remote_holder (Autodesk Fusion 360 design; units mm, degrees)
Autodesk Fusion 360 part; units mm, degrees
sketch "Sketch1" plane through (0, 0, 0) normal (0, 0, 1) x (1, 0, 0)
  line L0 (0, 0) -> (-42, 0)
  line L1 (-42, 0) -> (-42, 10)
  line L2 (-42, 10) -> (0, 10)
  line L3 (0, 10) -> (0, 0)
  line L4 (3.6, -3.6) -> (-45.6, -3.6)
  line L5 (-45.6, -3.6) -> (-45.6, 13.6)
  line L6 (-45.6, 13.6) -> (3.6, 13.6)
  line L7 (3.6, 13.6) -> (3.6, -3.6)
  dimension "d1" = 42
  dimension "d2" = 10
  dimension "d3" = -3.6
  constraint horizontal L0
  constraint vertical L1
  constraint horizontal L2
  constraint vertical L3
  constraint coincident L0.start L3.end
  measures "d1" distance of L0.start L0.end
  measures "d2" distance of L0.start L2.end
extrude "Extrude1" add sketch "Sketch1" along normal blind 65
extrude "Extrude2" add sketch "Sketch1" against normal blind 5 contours L0 L1 L2 L3 | L4 L5 L6 L7
sketch "Sketch2" plane through (0, -3.6, 0) normal (0, -1, 0) x (1, 0, 0)
  line L0 (3.6, -5) -> (3.6, 65)
  line L1 (3.6, 65) -> (-45.6, 65)
  line L2 (-45.6, 65) -> (-45.6, -5)
  line L3 (-45.6, -5) -> (3.6, -5)
  line L4 (0, 65, -3.6) -> (0, 65, 0)
  line L5 (-42, 65, -3.6) -> (-42, 65, 0)
  line L6 (-21, 65) -> (-21, -5)
  spline S0 degree 2 poles (-42, 65) (-21, 34) (0, 65) knots 0 0 0 5.982089 5.982089 5.982089 weights 1 2.19545 1
  point P0 (0, 65)
  point P1 (-42, 65)
  constraint coincident P0 S0.end
  constraint coincident L1 P0
  constraint coincident P1 S0.start
  constraint coincident L1 P1
  constraint midpoint L1 L6.start
  constraint midpoint L3 L6.end
extrude "Extrude3" cut sketch "Sketch2" against normal blind 13.6 contours L1 L6 S0 | L1 L6 S0
fillet "Fillet1" radius 4.5 3 edges at (-45.6, -3.6, 30) (-21, -3.6, -5) (3.6, -3.6, 30)
